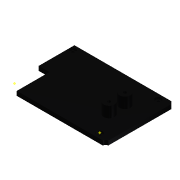
# Autodesk Inventor part: CustomBox_ardplate
Saved by Autodesk Inventor 2013 (Build 170138000, 138)
## iProperties
Created: 2013-03-21
Part Number: CustomBox_ardplate
Material: Generic
Document SubType Name: Modeling
Designer: Alexander
Density: 1 g/cm^3
Author: Alexander
Autodesk Inventor part; units mm, degrees
ref_plane "YZ Plane" through (0, 0, 0) normal (1, 0, 0) x (0, 1, 0)
ref_plane "XZ Plane" through (0, 0, 0) normal (0, 1, 0) x (-1, 0, 0)
ref_plane "XY Plane" through (0, 0, 0) normal (0, 0, 1) x (1, 0, 0)
sketch "Sketch1" plane through (0, 0, 0) normal (0, 1, 0) x (-1, 0, 0)
  line L0 (0, 0) -> (71.12, 0)
  line L1 (71.12, 0) -> (71.12, 40.64)
  line L2 (71.12, 40.64) -> (0, 40.64)
  line L3 (0, 40.64) -> (0, 0)
  dimension "d0" = 71.12
  dimension "d1" = 40.64
  constraints: 8 end point, 2 parallel, 1 horizontal, 1 perpendicular
  measures "d0" distance of L2.end L1.end
  measures "d1" distance of L0.end L1.end
extrude "Extrusion1" add sketch "Sketch1" along normal blind 2.54
sketch "Sketch8" plane through (0, 2.54, 0) normal (0, 1, 0) x (1, 0, 0)
  line L0 (0, -40.64) -> (0, 0) projected
  circle A0 centre (-6.35, -37.719) radius 0.8
  circle A1 centre (-6.35, -2.921) radius 0.8
  circle A2 centre (-57.15, -2.921) radius 0.8
  circle A3 centre (-57.15, -37.719) radius 0.8
  dimension "d75" = 1.6
  dimension "d76" = 1.6
  dimension "d77" = 1.6
  dimension "d78" = 1.6
  dimension "d79" = 6.35
  dimension "d108" = 50.8
  constraints: 4 centre point, 2 horizontal alignment, 2 vertical alignment
  measures "d75" diameter of A0
  measures "d76" diameter of A1
  measures "d77" diameter of A2
  measures "d78" diameter of A3
  measures "d79" distance from line of L0 A0.centre
  measures "d108" distance of A1.centre A2.centre
hole "Hole2" at (-57.15, 2.54, 2.921) at (-57.15, 2.54, 37.719) at (-6.35, 2.54, 37.719) at (-6.35, 2.54, 2.921) direction (0, -1, 0) diameter 1.6 end through all counterbore diameter 3.5 counterbore depth 1.27
sketch "Sketch9" plane through (0, 2.54, 0) normal (0, 1, 0) x (1, 0, 0)
  line L0 (0, 0) -> (-71.12, 0) projected
  line L1 (-71.12, 0) -> (-71.12, -40.64) projected
  line L2 (0, -40.64) -> (0, 0) projected
  arc A0 (0, -39.0525) -> (-1.5875, -40.64) centre (0, -40.64) ccw
  arc A1 (-1.5875, 0) -> (0, -1.5875) centre (0, 0) ccw
  arc A2 (-69.5325, -40.64) -> (-71.12, -39.0525) centre (-71.12, -40.64) ccw
  arc A3 (-71.12, -1.5875) -> (-69.5325, 0) centre (-71.12, 0) ccw
  line L3 (-1.5875, 0) -> (0, 0)
  line L4 (0, 0) -> (0, -1.5875)
  line L5 (0, -39.0525) -> (0, -40.64)
  line L6 (0, -40.64) -> (-1.5875, -40.64)
  line L7 (-69.5325, -40.64) -> (-71.12, -40.64)
  line L8 (-71.12, -40.64) -> (-71.12, -39.0525)
  line L9 (-69.5325, 0) -> (-71.12, 0)
  line L10 (-71.12, 0) -> (-71.12, -1.5875)
  point P0 (-69.85, -7.9375)
  dimension "d87" = 1.5875
  dimension "d89" = 1.5875
  dimension "d90" = 1.5875
  dimension "d91" = 1.5875
  constraints: 16 end point, 8 point on circle, 4 centre point, 4 coincident, 4 collinear, 2 point on line, 1 horizontal, 1 perpendicular, 1 vertical, 2 other
  measures "d87" radius of A0
  measures "d89" radius of A1
  measures "d90" radius of A2
  measures "d91" radius of A3
extrude "Extrusion9" cut sketch "Sketch9" against normal through all
sketch "Sketch10" plane through (0, 2.54, 0) normal (0, 1, 0) x (1, 0, 0)
  circle A0 centre (-13.4874, -15.5956) radius 3.175
  circle A1 centre (-13.4874, -25.0444) radius 3.175
  line L0 (0, -39.0525) -> (0, -1.5875) projected
  line L1 (-1.5875, 0) -> (-69.5325, 0) projected
  dimension "d95" = 6.35
  dimension "d96" = 6.35
  dimension "d122" = 13.4874
  dimension "d123" = 13.4874
  dimension "d125" = 9.4488
  dimension "d126" = 15.5956
  constraints: 2 centre point
  measures "d95" diameter of A0
  measures "d96" diameter of A1
  measures "d122" distance from line of L0 A0.centre
  measures "d123" distance from line of L0 A1.centre
  measures "d125" distance of A1.centre A0.centre
  measures "d126" distance from line of L1 A0.centre
extrude "Extrusion10" add sketch "Sketch10" along normal blind 6.35
sketch "Sketch11" plane through (-13.4874, 8.89, 15.5956) normal (0, 1, 0) x (1, 0, 0)
  circle A0 centre (0, 0) radius 3.175 projected
  circle A1 centre (0, -9.4488) radius 3.175 projected
  circle A2 centre (0, 0) radius 0.875
  circle A3 centre (0, -9.4488) radius 0.875
  line L0 (0, -12.6238) -> (17.5736, -12.6238)
  point P0 (13.4874, 15.5956)
  dimension "d106" = 1.75
  dimension "d107" = 1.75
  constraints: 2 centre point, 2 coincident, 2 end point, 2 horizontal, 1 vertical alignment, 1 other
  measures "d106" diameter of A2
  measures "d107" diameter of A3
sketch "Sketch12" plane through (0, 2.54, 0) normal (0, 1, 0) x (1, 0, 0)
  line L0 (-71.12, -1.5875) -> (-71.12, -39.0525) projected
  line L1 (-71.12, 2.2213) -> (-59.1056, 2.2213)
  line L2 (-59.1056, -41.9087) -> (-71.12, -41.9087)
  line L3 (-71.12, -41.9087) -> (-71.12, 2.2213)
  line L4 (0, -39.0525) -> (0, -1.5875) projected
  line L5 (-59.1056, -41.9087) -> (-52.7556, -41.9087)
  line L6 (-52.7556, -41.9087) -> (-52.7556, -21.2712)
  line L7 (-52.7556, -21.2712) -> (-59.1056, -21.2712)
  line L8 (-59.1056, 2.2213) -> (-59.1056, -21.2712)
  dimension "d128" = 20.6375
  dimension "d129" = 6.35
  constraints: 14 end point, 4 perpendicular, 2 parallel, 1 horizontal, 1 point on line
  measures "d128" distance of L5.end L6.end
  measures "d129" distance of L6.end L7.end
extrude "Extrusion11" cut sketch "Sketch12" against normal blind 25.4
extrude "Extrusion12" cut sketch "Sketch11" against normal blind 5 contours A2 | A3
body "Solid1"
